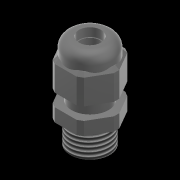
# Autodesk Inventor part: pg7_gland
Saved by Autodesk Inventor 2020.2 (Build 242310000, 310)
## iProperties
Created: 2020-04-23
Part Number: pg7_gland
Material: PC/ABS Plastic
Document SubType Name: Modeling
Designer: agmlego
Mass: 1.1539 g
Surface Area: 25.5096 cm^2
Volume: 3.22975 cm^3
Density: 0.357273 g/cm^3
Appearance: Smooth - Black
Author: agmlego
Autodesk Inventor part; units mm, degrees
ref_plane "YZ Plane" through (0, 0, 0) normal (1, 0, 0) x (0, 1, 0)
ref_plane "XZ Plane" through (0, 0, 0) normal (0, 1, 0) x (-1, 0, 0)
ref_plane "XY Plane" through (0, 0, 0) normal (0, 0, 1) x (1, 0, 0)
sketch "Sketch1" plane through (0, 0, 0) normal (0, 1, 0) x (-1, 0, 0)
  circle A0 centre (0, 0) radius 6.25
  dimension "d0" = 12.5
  constraints: 1 centre point, 1 coincident
  measures "d0" diameter of A0
extrude "Extrusion1" add sketch "Sketch1" along normal blind 8
sketch "Sketch2" plane through (0, 8, 0) normal (0, 1, 0) x (1, 0, 0)
  line L0 (-8.9489, 0) -> (-4.4745, 7.75)
  line L1 (-4.4745, 7.75) -> (4.4745, 7.75)
  line L2 (4.4745, 7.75) -> (8.9489, 0)
  line L3 (8.9489, 0) -> (4.4745, -7.75)
  line L4 (4.4745, -7.75) -> (-4.4745, -7.75)
  line L5 (-4.4745, -7.75) -> (-8.9489, 0)
  point P0 (0, 0)
  point P1 (0, 0)
  dimension "d3" = 15.5
  constraints: 12 end point, 1 coincident, 13 other
  measures "d3" distance between parallel lines of L1 L4
extrude "Extrusion2" add sketch "Sketch2" along normal blind 4.2
sketch "Sketch3" plane through (0, 12.2, 0) normal (0, 1, 0) x (1, 0, 0)
  circle A0 centre (0, 0) radius 5.875
  dimension "d6" = 11.75
  constraints: 1 centre point, 1 coincident
  measures "d6" diameter of A0
extrude "Extrusion3" add sketch "Sketch3" along normal blind 4
sketch "Sketch4" plane through (0, 16.2, 0) normal (0, 1, 0) x (1, 0, 0)
  line L0 (-4.4745, 7.75) -> (-8.9489, 0) projected
  line L1 (-8.9489, 0) -> (-4.4745, 7.75)
  line L2 (-4.4745, 7.75) -> (4.4745, 7.75)
  line L3 (4.4745, 7.75) -> (8.9489, 0)
  line L4 (8.9489, 0) -> (4.4745, -7.75)
  line L5 (4.4745, -7.75) -> (-4.4745, -7.75)
  line L6 (-4.4745, -7.75) -> (-8.9489, 0)
  point P0 (0, 0)
  point P1 (0, 0)
  constraints: 12 end point, 1 coincident, 13 other
extrude "Extrusion4" add sketch "Sketch4" along normal blind 8.9
sketch "Sketch5" plane through (0, 25.1, 0) normal (0, 1, 0) x (1, 0, 0)
  circle A0 centre (0, 0) radius 7.3
  dimension "d11" = 14.6
  constraints: 1 centre point, 1 coincident
  measures "d11" diameter of A0
extrude "Extrusion5" add sketch "Sketch5" along normal blind 4.5
fillet "Fillet1" radius 3 1 edges at (-7.3, 29.6, 0)
chamfer "Chamfer1" distance 1 angle 45 12 edges at (4.4745, 10.1, 7.75) (4.4745, 20.65, 7.75) (8.9489, 20.65, 0) (8.9489, 10.1, 0) (4.4745, 10.1, -7.75) (4.4745, 20.65, -7.75) (-4.4745, 10.1, -7.75) (-4.4745, 20.65, -7.75) (-8.9489, 10.1, 0) (-8.9489, 20.65, 0) (-4.4745, 20.65, 7.75) (-4.4745, 10.1, 7.75)
chamfer "Chamfer2" distance 1 angle 45 12 edges at (-4.2245, 25.1, 7.317) (-6.7117, 25.1, 3.875) (0, 25.1, 7.75) (6.7117, 25.1, 3.875) (4.2245, 25.1, 7.317) (8.4489, 25.1, 0) (6.7117, 25.1, -3.875) (4.2245, 25.1, -7.317) (0, 25.1, -7.75) (-4.2245, 25.1, -7.317) (-6.7117, 25.1, -3.875) (-8.4489, 25.1, 0)
thread "Thread1" size "G13.157x1.337" designation "G 1/4" class "A" standard "DIN Pipe Threads" full length
sketch "Sketch6" plane through (0, 0, 0) normal (0, -1, 0) x (1, 0, 0)
  circle A0 centre (0, 0) radius 6.25 projected
  constraints: 1 coincident
hole "Hole1" at (0, 0, 0) direction (0, 1, 0) diameter 8.8 depth 19.5
sketch "Sketch8" plane through (0, 29.6, 0) normal (0, 1, 0) x (1, 0, 0)
  circle A0 centre (0, 0) radius 4.3 projected
  constraints: 1 coincident
hole "Hole2" at (0, 29.6, 0) direction (0, -1, 0) diameter 7 depth 2.7
sketch "Sketch9" plane through (0, 26.9, 0) normal (0, 1, 0) x (1, 0, 0)
  circle A0 centre (0, 0) radius 3.5 projected
  constraints: 1 coincident
hole "Hole3" at (0, 26.9, 0) direction (0, -1, 0) diameter 6.4 end through all
body "Solid1"
